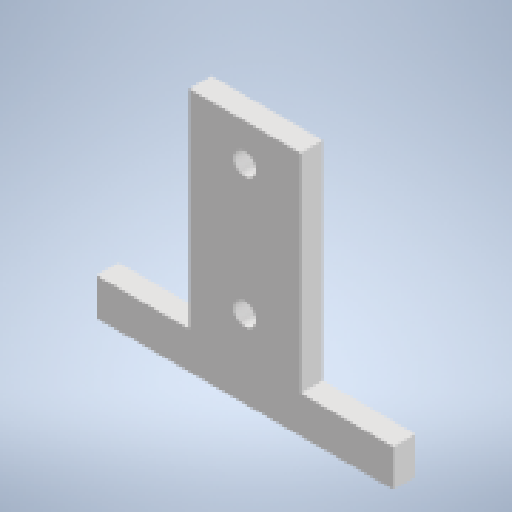
# Autodesk Inventor part: Soporte_Motorreductor
Saved by Autodesk Inventor 2024 (Build 280153000, 153)
## iProperties
Created: 2025-05-13
Part Number: Soporte_Motorreductor
Material: Genérico
Document SubType Name: Modeling
Designer: mario
Density: 1 g/cm^3
Appearance: Valor por defecto
Author: mario
Autodesk Inventor part; units mm, degrees
ref_plane "YZ Plane" through (0, 0, 0) normal (1, 0, 0) x (0, 1, 0)
ref_plane "XZ Plane" through (0, 0, 0) normal (0, 1, 0) x (-1, 0, 0)
ref_plane "XY Plane" through (0, 0, 0) normal (0, 0, 1) x (1, 0, 0)
sketch "Boceto1" plane through (0, 0, 0) normal (0, 0, 1) x (1, 0, 0)
  line L0 (-7.5, -16.5) -> (7.5, -16.5)
  line L1 (7.5, -16.5) -> (7.5, 16.5)
  line L2 (7.5, 16.5) -> (-7.5, 16.5)
  line L3 (-7.5, 16.5) -> (-7.5, -16.5)
  line L4 (-7.5, -16.5) -> (7.5, 16.5) construction
  line L5 (7.5, -16.5) -> (-7.5, 16.5) construction
  point P0 (0, 0)
  dimension "d7" = 33
  dimension "d8" = 15
  constraints: 12 end point, 2 midpoint, 2 parallel, 1 horizontal, 1 perpendicular
  measures "d7" distance of L0.end L1.end
  measures "d8" distance of L0.start L0.end
extrude "Extrusión1" add sketch "Boceto1" along normal blind 3
sketch "Boceto2" plane through (0, 0, 0) normal (0, 0, -1) x (-1, 0, 0)
  line L0 (-20, -16.5) -> (20, -16.5)
  line L1 (20, -16.5) -> (20, -11.5)
  line L2 (20, -11.5) -> (-20, -11.5)
  line L3 (-20, -11.5) -> (-20, -16.5)
  point P0 (0, 0)
  point P1 (7.5, -16.5)
  dimension "d2" = 20
  dimension "d3" = 20
  dimension "d4" = 5
  constraints: 8 end point, 2 parallel, 1 horizontal, 1 perpendicular, 1 point on line
  measures "d2" distance from line of point (0, 0) L3
  measures "d3" distance from line of L1 point (0, 0)
  measures "d4" distance of L0.end L1.end
extrude "Extrusión2" add sketch "Boceto2" against normal blind 3
sketch "Boceto3" plane through (0, 0, 0) normal (0, 0, -1) x (-1, 0, 0)
  line L0 (-20, -16.5) -> (20, -16.5) construction
  point P0 (0, 0)
  point P1 (0, -6)
  point P2 (0, 11.5)
  dimension "d9" = 10.5
  dimension "d10" = 17.5
  measures "d9" distance from line of L0 point (0, -6)
  measures "d10" distance of point (0, -6) point (0, 11.5)
hole "Agujero1" at (0, -6, 0) at (0, 11.5, 0) direction (0, 0, 1) diameter 3 end through all
